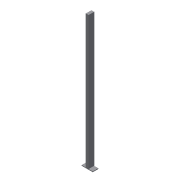
# Autodesk Inventor part: Lift Towers
Saved by Autodesk Inventor 2015 (Build 190159000, 159)
## iProperties
Created: 2015-03-07
Part Number: Lift Towers
Material: Generic
Document SubType Name: Modeling
Designer: Jaden
Density: 1 g/cm^3
Appearance: Default
Author: Jaden
Autodesk Inventor part; units mm, degrees
ref_plane "YZ Plane" through (0, 0, 0) normal (1, 0, 0) x (0, 1, 0)
ref_plane "XZ Plane" through (0, 0, 0) normal (0, 1, 0) x (-1, 0, 0)
ref_plane "XY Plane" through (0, 0, 0) normal (0, 0, 1) x (1, 0, 0)
sketch "Sketch3" plane through (0, 0, 0) normal (0, 0, 1) x (1, 0, 0)
  line L0 (0, 0) -> (101.6, 0)
  line L1 (101.6, 0) -> (101.6, 6.35)
  line L2 (101.6, 6.35) -> (63.5, 6.35)
  line L3 (101.6, 6.35) -> (139.7, 6.35) construction
  line L4 (63.5, 6.35) -> (63.5, 1225.55)
  line L5 (63.5, 1225.55) -> (38.1, 1225.55)
  line L6 (38.1, 1225.55) -> (38.1, 6.35)
  line L7 (38.1, 6.35) -> (0, 6.35)
  line L8 (0, 6.35) -> (0, 0)
  dimension "d15" = 101.6
  dimension "d16" = 6.35
  dimension "d17" = 38.1
  dimension "d18" = 180
  dimension "d19" = 1219.2
  dimension "d20" = 90
  dimension "d21" = 25.4
  dimension "d22" = 1219.2
  dimension "d23" = 90
  constraints: 18 end point, 4 perpendicular, 3 horizontal, 1 collinear, 1 parallel, 1 point on line
  measures "d15" distance of L0.start L0.end
  measures "d16" distance of L0.end L1.end
  measures "d17" distance of L1.end L2.end
  measures "d18" angle of L2 L3
  measures "d19" distance of L2.end L4.end
  measures "d20" angle of L2 L4
  measures "d21" distance of L4.end L5.end
  measures "d22" distance of L5.end L6.end
  measures "d23" angle of L6 L5
extrude "Extrusion3" add sketch "Sketch3" along normal blind 50.8
body "Solid3"
